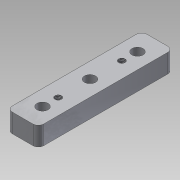
# Autodesk Inventor part: VSlot Spacer Block
Saved by Autodesk Inventor 2013 SP2 (Build 170200200, 200)
## iProperties
Created: 2013-06-30
Part Number: VSlot Spacer Block
Material: Aluminum 6061
Document SubType Name: Modeling
Designer: Jon Hollander
Density: 2.71 g/cm^3
Mass: 50.866 g
Surface Area: 67.2324 cm^2
Volume: 18.7698 cm^3
Author: Jon Hollander
Autodesk Inventor part; units mm, degrees
ref_plane "YZ Plane" through (0, 0, 0) normal (1, 0, 0) x (0, 1, 0)
ref_plane "XZ Plane" through (0, 0, 0) normal (0, 1, 0) x (-1, 0, 0)
ref_plane "XY Plane" through (0, 0, 0) normal (0, 0, 1) x (1, 0, 0)
sketch "Sketch1" plane through (0, 0, 0) normal (0, 0, 1) x (1, 0, 0)
  line L0 (-10, -43.02) -> (10, -43.02)
  line L1 (10, -43.02) -> (10, 43.02)
  line L2 (10, 43.02) -> (-10, 43.02)
  line L3 (-10, 43.02) -> (-10, -43.02)
  line L4 (-10, -43.02) -> (10, 43.02) construction
  line L5 (10, -43.02) -> (-10, 43.02) construction
  point P0 (0, 0)
  dimension "d0" = 20
  dimension "d1" = 86.04
  constraints: 12 end point, 2 midpoint, 2 parallel, 1 horizontal, 1 perpendicular
  measures "d0" distance of L2.end L1.end
  measures "d1" distance of L1.end L0.end
extrude "Extrusion1" add sketch "Sketch1" along normal blind 12
sketch "Sketch2" plane through (0, 0, 12) normal (0, 0, 1) x (1, 0, 0)
  point P0 (0, 0)
  point P1 (0, 0)
  point P2 (0, 30.32)
  point P3 (0, -30.32)
  dimension "d4" = 30.32
  dimension "d5" = 30.32
  constraints: 1 coincident
  measures "d4" distance of point (0, 0) point (0, 30.32)
  measures "d5" distance of point (0, -30.32) point (0, 0)
hole "Hole1" at (0, 0, 12) at (0, 30.32, 12) at (0, -30.32, 12) direction (0, 0, -1) diameter 7.14 end through all
sketch "Sketch3" plane through (0, 0, 12) normal (0, 0, 1) x (1, 0, 0)
  circle A0 centre (0, 0) radius 3.57 projected
  point P0 (0, 20.32)
  point P1 (0, -20.32)
  dimension "d13" = 20.32
  dimension "d14" = 20.32
  measures "d13" distance of A0.centre point (0, -20.32)
  measures "d14" distance of point (0, 20.32) A0.centre
hole "Hole2" at (0, 20.32, 12) at (0, -20.32, 12) direction (0, 0, -1) diameter 4.134 end through all thread size "M5x0.8" class "6H" standard "ANSI Metric M Profile"
fillet "Fillet1" radius 3.36 4 edges at (10, 43.02, 6) (-10, 43.02, 6) (10, -43.02, 6) (-10, -43.02, 6)
equation "\"d5\" = d4"
equation "\"d14\" = d13"
body "Solid1"
